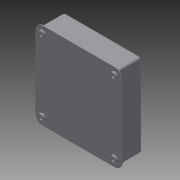
# Autodesk Inventor part: BRIX
Saved by Autodesk Inventor 2013 (Build 170138000, 138)
## iProperties
Created: 2014-05-15
Part Number: BRIX
Material: 一般
Document SubType Name: Modeling
Designer: andou
Density: 1 g/cm^3
Author: andou
Autodesk Inventor part; units mm, degrees
ref_plane "YZ Plane" through (0, 0, 0) normal (1, 0, 0) x (0, 1, 0)
ref_plane "XZ Plane" through (0, 0, 0) normal (0, 1, 0) x (-1, 0, 0)
ref_plane "XY Plane" through (0, 0, 0) normal (0, 0, 1) x (1, 0, 0)
sketch "スケッチ1" plane through (0, 0, 0) normal (0, 1, 0) x (-1, 0, 0)
  line L0 (-60, 60) -> (60, 60)
  line L1 (60, 60) -> (60, -60)
  line L2 (60, -60) -> (-60, -60)
  line L3 (-60, -60) -> (-60, 60)
  point P0 (0, 0)
  dimension "d0" = 120
  dimension "d2" = 120
  dimension "d3" = 60
  dimension "d4" = 60
  constraints: 8 end point, 2 parallel, 1 horizontal, 1 perpendicular
  measures "d0" distance of L0.start L0.end
  measures "d2" distance of L2.end L0.start
  measures "d3" distance from line of L0 point (0, 0)
  measures "d4" distance from line of L1 point (0, 0)
extrude "押し出し1" add sketch "スケッチ1" along normal blind 1
sketch "スケッチ2" plane through (0, 0, 0) normal (0, -1, 0) x (1, 0, 0)
  circle A0 centre (-50, 50) radius 2
  circle A1 centre (50, 50) radius 2
  circle A2 centre (-50, -50) radius 2
  circle A3 centre (50, -50) radius 2
  circle A4 centre (-50, 50) radius 5
  circle A5 centre (50, 50) radius 5
  circle A6 centre (50, -50) radius 5
  circle A7 centre (-50, -50) radius 5
  point P0 (0, 0)
  dimension "d7" = 4
  dimension "d9" = 100
  dimension "d10" = 100
  dimension "d11" = 100
  dimension "d12" = 100
  dimension "d13" = 50
  dimension "d14" = 50
  dimension "d15" = 50
  dimension "d16" = 50
  dimension "d17" = 10
  constraints: 8 centre point, 6 equal radius, 4 coincident
  measures "d7" diameter of A0
  measures "d9" distance of A1.centre A0.centre
  measures "d10" distance of A3.centre A2.centre
  measures "d11" distance of A0.centre A2.centre
  measures "d12" distance of A1.centre A3.centre
  measures "d13" horizontal distance of point (0, 0) A2.centre
  measures "d14" horizontal distance of A3.centre point (0, 0)
  measures "d15" horizontal distance of point (0, 0) A2.centre
  measures "d16" horizontal distance of A1.centre point (0, 0)
  measures "d17" diameter of A4
extrude "押し出し2" add sketch "スケッチ2" along normal blind 3
sketch "スケッチ3" plane through (50, 0, 50) normal (0, -1, 0) x (1, 0, 0)
  circle A0 centre (0, 0) radius 2 projected
  circle A1 centre (0, -100) radius 2 projected
  circle A2 centre (0, -100) radius 5 projected
  circle A3 centre (-100, 0) radius 2 projected
  circle A4 centre (-100, 0) radius 5 projected
  circle A5 centre (0, 0) radius 2 projected
  circle A6 centre (0, 0) radius 5 projected
  circle A7 centre (-100, -100) radius 2 projected
  circle A8 centre (-100, -100) radius 5 projected
  line L0 (-110, -110) -> (-110, 10) projected
  line L1 (-110, 10) -> (10, 10) projected
  line L2 (10, 10) -> (10, -110) projected
  line L3 (10, -110) -> (-110, -110) projected
  point P0 (-50, -50)
hole "穴1" at (50, 0, 50) at (-50, 0, 50) at (-50, 0, -50) at (50, 0, -50) direction (0, 1, 0) diameter 4 end through all
fillet "フィレット1" radius 10 4 edges at (-60, 0.5, 60) (60, 0.5, 60) (-60, 0.5, -60) (60, 0.5, -60)
sketch "スケッチ4" plane through (0, 1, 0) normal (0, 1, 0) x (1, 0, 0)
  line L0 (-54, 57.5) -> (54, 57.5)
  line L1 (54, 57.5) -> (54, -57.5)
  line L2 (54, -57.5) -> (-54, -57.5)
  line L3 (-54, -57.5) -> (-54, 57.5)
  point P0 (0, 0)
  dimension "d28" = 115
  dimension "d31" = 108
  dimension "d32" = 54
  dimension "d33" = 57.5
  constraints: 8 end point, 2 parallel, 1 horizontal, 1 perpendicular
  measures "d28" distance of L2.end L0.start
  measures "d31" distance of L0.start L0.end
  measures "d32" distance from line of L1 point (0, 0)
  measures "d33" distance from line of L0 point (0, 0)
extrude "押し出し3" add sketch "スケッチ4" along normal blind 33
fillet "フィレット2" radius 3 8 edges at (54, 34, 0) (54, 17.5, 57.5) (0, 34, 57.5) (-54, 34, 0) (0, 34, -57.5) (54, 17.5, -57.5) (-54, 17.5, -57.5) (-54, 17.5, 57.5)
sketch "スケッチ5" plane through (0, 34, 0) normal (0, 1, 0) x (1, 0, 0)
  circle A0 centre (39, -36.5) radius 4.5
  line L0 (-51, -57.5) -> (51, -57.5) projected
  line L1 (54, -54.5) -> (54, 54.5) projected
  line L2 (51, 54.5) -> (-51, 54.5) projected
  line L3 (-51, 54.5) -> (-51, -54.5) projected
  line L4 (-51, -54.5) -> (51, -54.5) projected
  line L5 (51, -54.5) -> (51, 54.5) projected
  line L6 (-42.1313, 44.6736) -> (-3.3859, 44.6736) construction
  line L7 (-3.3859, 44.6736) -> (-3.3859, 38.3462) construction
  line L8 (-3.3859, 38.3462) -> (-42.1313, 38.3462) construction
  line L9 (-42.1313, 38.3462) -> (-42.1313, 44.6736) construction
  spline S0 degree 2 poles (-37.4392, 39.86) (-37.7674, 39.7263) (-38.8168, 39.471) (-39.3274, 39.471) knots 0 0 0 1 2 2 2
  spline S1 degree 2 poles (-39.3274, 39.471) (-40.5065, 39.471) (-41.9044, 40.8325) (-41.9044, 42.0804) knots 0 0 0 1 2 2 2
  spline S2 degree 2 poles (-41.9044, 42.0804) (-41.9044, 43.2555) (-40.5065, 44.6736) (-39.2909, 44.6736) knots 0 0 0 1 2 2 2
  spline S3 degree 2 poles (-39.2909, 44.6736) (-38.6629, 44.6736) (-37.8768, 44.4346) (-37.4595, 44.232) knots 0 0 0 1 2 2 2
  line L10 (-37.4595, 44.232) -> (-37.4595, 43.0569)
  line L11 (-37.4595, 43.0569) -> (-37.5729, 43.0569)
  spline S4 degree 2 poles (-37.5729, 43.0569) (-37.6621, 43.1258) (-38.0024, 43.3892) (-38.1645, 43.4783) knots 0 0 0 1 2 2 2
  spline S5 degree 2 poles (-38.1645, 43.4783) (-38.3509, 43.5877) (-38.8452, 43.7417) (-39.1207, 43.7417) knots 0 0 0 1 2 2 2
  spline S6 degree 2 poles (-39.1207, 43.7417) (-39.4408, 43.7417) (-39.9716, 43.5391) (-40.1783, 43.3325) knots 0 0 0 1 2 2 2
  spline S7 degree 2 poles (-40.1783, 43.3325) (-40.3768, 43.1299) (-40.6078, 42.5099) (-40.6078, 42.1007) knots 0 0 0 1 2 2 2
  spline S8 degree 2 poles (-40.6078, 42.1007) (-40.6078, 41.2255) (-39.7285, 40.3908) (-38.9708, 40.3908) knots 0 0 0 1 2 2 2
  spline S9 degree 2 poles (-38.9708, 40.3908) (-38.9019, 40.3908) (-38.7236, 40.3989) (-38.6548, 40.403) knots 0 0 0 1 2 2 2
  line L12 (-38.6548, 40.403) -> (-38.6548, 41.3876)
  line L13 (-38.6548, 41.3876) -> (-39.6232, 41.3876)
  line L14 (-39.6232, 41.3876) -> (-39.6232, 42.3235)
  line L15 (-39.6232, 42.3235) -> (-37.4392, 42.3235)
  line L16 (-37.4392, 42.3235) -> (-37.4392, 39.86)
  line L17 (-34.0032, 39.5764) -> (-36.6937, 39.5764)
  line L18 (-36.6937, 39.5764) -> (-36.6937, 40.4475)
  line L19 (-36.6937, 40.4475) -> (-35.9765, 40.4475)
  line L20 (-35.9765, 40.4475) -> (-35.9765, 43.7052)
  line L21 (-35.9765, 43.7052) -> (-36.6937, 43.7052)
  line L22 (-36.6937, 43.7052) -> (-36.6937, 44.5764)
  line L23 (-36.6937, 44.5764) -> (-34.0032, 44.5764)
  line L24 (-34.0032, 44.5764) -> (-34.0032, 43.7052)
  line L25 (-34.0032, 43.7052) -> (-34.7204, 43.7052)
  line L26 (-34.7204, 43.7052) -> (-34.7204, 40.4475)
  line L27 (-34.7204, 40.4475) -> (-34.0032, 40.4475)
  line L28 (-34.0032, 40.4475) -> (-34.0032, 39.5764)
  spline S10 degree 2 poles (-28.9951, 39.86) (-29.3233, 39.7263) (-30.3728, 39.471) (-30.8833, 39.471) knots 0 0 0 1 2 2 2
  spline S11 degree 2 poles (-30.8833, 39.471) (-32.0624, 39.471) (-33.4603, 40.8325) (-33.4603, 42.0804) knots 0 0 0 1 2 2 2
  spline S12 degree 2 poles (-33.4603, 42.0804) (-33.4603, 43.2555) (-32.0624, 44.6736) (-30.8468, 44.6736) knots 0 0 0 1 2 2 2
  spline S13 degree 2 poles (-30.8468, 44.6736) (-30.2188, 44.6736) (-29.4327, 44.4346) (-29.0154, 44.232) knots 0 0 0 1 2 2 2
  line L29 (-29.0154, 44.232) -> (-29.0154, 43.0569)
  line L30 (-29.0154, 43.0569) -> (-29.1288, 43.0569)
  spline S14 degree 2 poles (-29.1288, 43.0569) (-29.218, 43.1258) (-29.5583, 43.3892) (-29.7204, 43.4783) knots 0 0 0 1 2 2 2
  spline S15 degree 2 poles (-29.7204, 43.4783) (-29.9068, 43.5877) (-30.4011, 43.7417) (-30.6766, 43.7417) knots 0 0 0 1 2 2 2
  spline S16 degree 2 poles (-30.6766, 43.7417) (-30.9967, 43.7417) (-31.5275, 43.5391) (-31.7342, 43.3325) knots 0 0 0 1 2 2 2
  spline S17 degree 2 poles (-31.7342, 43.3325) (-31.9327, 43.1299) (-32.1637, 42.5099) (-32.1637, 42.1007) knots 0 0 0 1 2 2 2
  spline S18 degree 2 poles (-32.1637, 42.1007) (-32.1637, 41.2255) (-31.2844, 40.3908) (-30.5267, 40.3908) knots 0 0 0 1 2 2 2
  spline S19 degree 2 poles (-30.5267, 40.3908) (-30.4578, 40.3908) (-30.2796, 40.3989) (-30.2107, 40.403) knots 0 0 0 1 2 2 2
  line L31 (-30.2107, 40.403) -> (-30.2107, 41.3876)
  line L32 (-30.2107, 41.3876) -> (-31.1791, 41.3876)
  line L33 (-31.1791, 41.3876) -> (-31.1791, 42.3235)
  line L34 (-31.1791, 42.3235) -> (-28.9951, 42.3235)
  line L35 (-28.9951, 42.3235) -> (-28.9951, 39.86)
  line L36 (-28.5859, 39.5764) -> (-26.8963, 44.5764)
  line L37 (-26.8963, 44.5764) -> (-25.5267, 44.5764)
  line L38 (-25.5267, 44.5764) -> (-23.8371, 39.5764)
  line L39 (-23.8371, 39.5764) -> (-25.1296, 39.5764)
  line L40 (-25.1296, 39.5764) -> (-25.4416, 40.5974)
  line L41 (-25.4416, 40.5974) -> (-27.0138, 40.5974)
  line L42 (-27.0138, 40.5974) -> (-27.3298, 39.5764)
  line L43 (-27.3298, 39.5764) -> (-28.5859, 39.5764)
  line L44 (-25.7172, 41.5051) -> (-26.2277, 43.1582)
  line L45 (-26.2277, 43.1582) -> (-26.7423, 41.5051)
  line L46 (-26.7423, 41.5051) -> (-25.7172, 41.5051)
  spline S20 degree 2 poles (-19.3436, 41.108) (-19.3436, 40.7352) (-19.6272, 40.172) (-19.8622, 39.9856) knots 0 0 0 1 2 2 2
  spline S21 degree 2 poles (-19.8622, 39.9856) (-20.1459, 39.7628) (-20.8185, 39.5764) (-21.3412, 39.5764) knots 0 0 0 1 2 2 2
  line L47 (-21.3412, 39.5764) -> (-23.3387, 39.5764)
  line L48 (-23.3387, 39.5764) -> (-23.3387, 44.5764)
  line L49 (-23.3387, 44.5764) -> (-21.5762, 44.5764)
  spline S22 degree 2 poles (-21.5762, 44.5764) (-21.0251, 44.5764) (-20.4578, 44.4913) (-20.2107, 44.3576) knots 0 0 0 1 2 2 2
  spline S23 degree 2 poles (-20.2107, 44.3576) (-19.9392, 44.2158) (-19.6758, 43.7295) (-19.6758, 43.4135) knots 0 0 0 1 2 2 2
  spline S24 degree 2 poles (-19.6758, 43.4135) (-19.6758, 43.0488) (-20.0405, 42.4775) (-20.3647, 42.3438) knots 0 0 0 1 2 2 2
  line L50 (-20.3647, 42.3438) -> (-20.3647, 42.3195)
  spline S25 degree 2 poles (-20.3647, 42.3195) (-19.8987, 42.2222) (-19.3436, 41.6185) (-19.3436, 41.108) knots 0 0 0 1 2 2 2
  spline S26 degree 2 poles (-20.6402, 41.1282) (-20.6402, 41.3632) (-20.8266, 41.6266) (-21.013, 41.6955) knots 0 0 0 1 2 2 2
  spline S27 degree 2 poles (-21.013, 41.6955) (-21.1264, 41.7401) (-21.5275, 41.7482) (-21.8598, 41.7482) knots 0 0 0 1 2 2 2
  line L51 (-21.8598, 41.7482) -> (-22.0907, 41.7482)
  line L52 (-22.0907, 41.7482) -> (-22.0907, 40.488)
  line L53 (-22.0907, 40.488) -> (-22.0219, 40.488)
  spline S28 degree 2 poles (-22.0219, 40.488) (-21.5356, 40.488) (-21.1629, 40.5002) (-20.9684, 40.5853) knots 0 0 0 1 2 2 2
  spline S29 degree 2 poles (-20.9684, 40.5853) (-20.7982, 40.6623) (-20.6402, 40.9459) (-20.6402, 41.1282) knots 0 0 0 1 2 2 2
  spline S30 degree 2 poles (-20.9522, 43.1663) (-20.9522, 43.2879) (-21.0778, 43.5431) (-21.2074, 43.5999) knots 0 0 0 1 2 2 2
  spline S31 degree 2 poles (-21.2074, 43.5999) (-21.329, 43.6566) (-21.6694, 43.6647) (-22.0057, 43.6647) knots 0 0 0 1 2 2 2
  line L54 (-22.0057, 43.6647) -> (-22.0907, 43.6647)
  line L55 (-22.0907, 43.6647) -> (-22.0907, 42.6031)
  line L56 (-22.0907, 42.6031) -> (-21.9327, 42.6031)
  spline S32 degree 2 poles (-21.9327, 42.6031) (-21.6126, 42.6031) (-21.3533, 42.6153) (-21.2155, 42.6801) knots 0 0 0 1 2 2 2
  spline S33 degree 2 poles (-21.2155, 42.6801) (-21.0656, 42.753) (-20.9522, 43.0002) (-20.9522, 43.1663) knots 0 0 0 1 2 2 2
  line L57 (-14.4651, 44.5764) -> (-16.1912, 41.6631)
  line L58 (-16.1912, 41.6631) -> (-16.1912, 39.5764)
  line L59 (-16.1912, 39.5764) -> (-17.4473, 39.5764)
  line L60 (-17.4473, 39.5764) -> (-17.4473, 41.6023)
  line L61 (-17.4473, 41.6023) -> (-19.2018, 44.5764)
  line L62 (-19.2018, 44.5764) -> (-17.7715, 44.5764)
  line L63 (-17.7715, 44.5764) -> (-16.795, 42.7936)
  line L64 (-16.795, 42.7936) -> (-15.8509, 44.5764)
  line L65 (-15.8509, 44.5764) -> (-14.4651, 44.5764)
  line L66 (-13.051, 39.5764) -> (-13.051, 43.6242)
  line L67 (-13.051, 43.6242) -> (-14.53, 43.6242)
  line L68 (-14.53, 43.6242) -> (-14.53, 44.5764)
  line L69 (-14.53, 44.5764) -> (-10.316, 44.5764)
  line L70 (-10.316, 44.5764) -> (-10.316, 43.6242)
  line L71 (-10.316, 43.6242) -> (-11.795, 43.6242)
  line L72 (-11.795, 43.6242) -> (-11.795, 39.5764)
  line L73 (-11.795, 39.5764) -> (-13.051, 39.5764)
  line L74 (-9.8014, 39.5764) -> (-9.8014, 44.5764)
  line L75 (-9.8014, 44.5764) -> (-6.4222, 44.5764)
  line L76 (-6.4222, 44.5764) -> (-6.4222, 43.6242)
  line L77 (-6.4222, 43.6242) -> (-8.5535, 43.6242)
  line L78 (-8.5535, 43.6242) -> (-8.5535, 42.7449)
  line L79 (-8.5535, 42.7449) -> (-6.5883, 42.7449)
  line L80 (-6.5883, 42.7449) -> (-6.5883, 41.7927)
  line L81 (-6.5883, 41.7927) -> (-8.5535, 41.7927)
  line L82 (-8.5535, 41.7927) -> (-8.5535, 40.5286)
  line L83 (-8.5535, 40.5286) -> (-6.4222, 40.5286)
  line L84 (-6.4222, 40.5286) -> (-6.4222, 39.5764)
  line L85 (-6.4222, 39.5764) -> (-9.8014, 39.5764)
  point P0 (0, 0)
  dimension "d37" = 9
  dimension "d39" = 21
  dimension "d40" = 15
  constraints: 1 centre point, 2 other
  measures "d37" diameter of A0
  measures "d39" distance from line of A0.centre L0
  measures "d40" distance from line of A0.centre L1
extrude "押し出し4" cut sketch "スケッチ5" against normal blind 0.5 contours A0 | S0 S1 S2 S3 L10 L11 S4 S5 S6 S7 S8 S9 L12 L13 L14 L15 L16 | L17 L18 L19 L20 L21 L22 L23 L24 L25 L26 L27 L28 | S10 S11 S12 S13 L29 L30 S14 S15 S16 S17 S18 S19 L31 L32 L33 L34 L35 | L36 L37 L38 L39 L40 L41 L42 L43 | S20 S21 L47 L48 L49 S22 S23 S24 L50 S25 | L69 L70 L71 L72 L73 L66 L67 L68 L57 | L57 L68 L65 | L57 L58 L59 L60 L61 L62 L63 L64 L65 L68 | L74 L75 L76 L77 L78 L79 L80 L81 L82 L83 L84 L85
chamfer "面取り1" distance 3 distance2 0.5 1 edges at (34.5, 34, 36.5) measured on face at (34, 34, 36.5)
